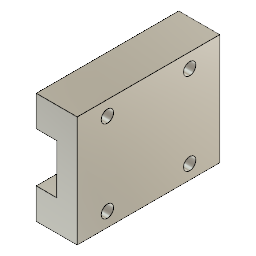
_mock linear rail carriage 12MM.53e73ab0-8921-47f2-a0a6-a6fb6bb4431b (Autodesk Fusion 360 design; units mm, degrees)
Autodesk Fusion 360 part; units mm, degrees
note: some values were not read from the file. Set by a fixed rule: which sketch regions a step uses.
sketch "Sketch1" plane through (0, 0, 0) normal (0, 1, 0) x (1, 0, 0)
  line L0 (0, 0) -> (10, 0)
  line L1 (10, 0) -> (10, -27)
  line L2 (10, -27) -> (0, -27)
  line L3 (0, -27) -> (0, 0)
  line L4 (0, -19.5) -> (5, -19.5)
  line L5 (5, -19.5) -> (5, -7.5)
  line L6 (5, -7.5) -> (0, -7.5)
  line L7 (0, -7.5) -> (0, -19.5)
  dimension "d1" = 10
  dimension "d2" = 27
  dimension "d3" = 12
  dimension "d4" = 5
  dimension "d6" = 7.5
  measures "d1" distance of L0.start
  measures "d6" distance of L0 L6
extrude "Extrude1" add sketch "Sketch1" along normal blind 34.7 contours L0 L1 L2 L3 L4 L5 L6
sketch "Sketch2" plane through (10, 0, 0) normal (1, 0, 0) x (0, 1, 0)
  line L0 (0, 27) -> (0, 0)
  line L1 (0, 0) -> (34.7, 0)
  line L2 (34.7, 0) -> (34.7, 27)
  line L3 (34.7, 27) -> (0, 27)
  line L4 (7.35, 3.5) -> (27.35, 3.5)
  line L5 (27.35, 3.5) -> (27.35, 23.5)
  line L6 (27.35, 23.5) -> (7.35, 23.5)
  line L7 (7.35, 23.5) -> (7.35, 3.5)
  circle A0 centre (7.35, 23.5) radius 1.5
  circle A1 centre (27.35, 23.5) radius 1.5
  circle A2 centre (7.35, 3.5) radius 1.5
  circle A3 centre (27.35, 3.5) radius 1.5
  dimension "d9" = 20
  dimension "d10" = 20
  dimension "d11" = 3.5
  dimension "d12" = 7.35
  dimension "d13" = 3
  dimension "d14" = 3
  dimension "d15" = 3
  dimension "d16" = 3
  measures "d11" distance of L3 L6
  measures "d12" distance of L0 L7
  measures "d13" diameter of A0
  measures "d14" diameter of A1
  measures "d15" diameter of A2
  measures "d16" diameter of A3
extrude "Extrude2" cut sketch "Sketch2" against normal blind 5 contours L4 L7 A2 | L4 L7 A2 | L4 L5 A3 | L4 L5 A3 | L6 L7 A0 | L6 L7 A0 | L5 L6 A1 | L5 L6 A1
equation "d12 = 9.85 mm - 2.5 mm"
